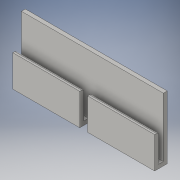
# Autodesk Inventor part: Handles
Saved by Autodesk Inventor 2016 (Build 200138000, 138)
## iProperties
Created: 2017-03-11
Part Number: Handles
Material: Generic
Document SubType Name: Modeling
Designer: RoboticsUser
Density: 1 g/cm^3
Appearance: Default
Author: RoboticsUser
Autodesk Inventor part; units mm, degrees
ref_plane "YZ Plane" through (0, 0, 0) normal (1, 0, 0) x (0, 1, 0)
ref_plane "XZ Plane" through (0, 0, 0) normal (0, 1, 0) x (-1, 0, 0)
ref_plane "XY Plane" through (0, 0, 0) normal (0, 0, 1) x (1, 0, 0)
sketch "Sketch5" plane through (0, 0, 0) normal (1, 0, 0) x (0, 1, 0)
  line L0 (0, 0) -> (101.6, 0)
  line L1 (101.6, 0) -> (101.6, -20.32)
  line L2 (101.6, -20.32) -> (0, -20.32)
  line L3 (0, -20.32) -> (0, 0)
  line L4 (101.6, -6.35) -> (6.35, -6.35)
  line L5 (6.35, -6.35) -> (6.35, -13.97)
  line L6 (6.35, -13.97) -> (101.6, -13.97)
  line L7 (101.6, -13.97) -> (101.6, -6.35)
  line L8 (101.6, 0) -> (50.8, 0)
  line L9 (50.8, -6.35) -> (101.6, -6.35)
  line L10 (101.6, -6.35) -> (101.6, 0)
  dimension "d26" = 101.6
  dimension "d27" = 20.32
  dimension "d28" = 95.25
  dimension "d29" = 7.62
  dimension "d30" = 6.35
  dimension "d31" = 50.8
  constraints: 22 end point, 5 parallel, 3 horizontal, 2 perpendicular, 2 point on line
  measures "d26" distance of L1.end L2.end
  measures "d27" distance of L0.end L1.end
  measures "d28" distance of L6.end L5.end
  measures "d29" distance of L4.end L5.end
  measures "d30" distance between parallel lines of L0 L4
  measures "d31" distance of L9.end L9.start
extrude "Extrusion4" add sketch "Sketch5" against normal blind 228.6
sketch "Sketch6" plane through (0, 0, 0) normal (1, 0, 0) x (0, 0, -1)
  line L0 (0, 101.6) -> (0, 0) projected
  line L1 (20.32, 0) -> (20.32, 101.6) projected
  line L2 (20.32, 101.6) -> (0, 101.6) projected
  line L3 (0, 0) -> (20.32, 0) projected
  line L4 (0, 101.6) -> (20.32, 101.6) projected
  line L5 (13.97, 101.6) -> (6.35, 101.6)
  line L6 (6.35, 101.6) -> (6.35, 6.35)
  line L7 (6.35, 6.35) -> (13.97, 6.35)
  line L8 (13.97, 6.35) -> (13.97, 101.6)
  line L9 (0, 0) -> (0, 101.6) projected
  line L10 (0, 101.6) -> (6.35, 101.6)
  line L11 (6.35, 101.6) -> (6.35, 50.8)
  line L12 (6.35, 50.8) -> (0, 50.8)
  line L13 (0, 50.8) -> (0, 101.6)
  dimension "d34" = 7.62
  dimension "d35" = 95.25
  dimension "d36" = 6.35
  dimension "d37" = 50.8
  constraints: 16 end point, 4 parallel, 2 horizontal, 2 perpendicular, 2 point on line
  measures "d34" distance of L7.end L6.end
  measures "d35" distance of L6.end L5.end
  measures "d36" distance between parallel lines of L0 L6
  measures "d37" distance between parallel lines of L3 L12
extrude "Extrusion5" cut sketch "Sketch6" against normal blind 228.6 contours L2 L8 L7 L6
sketch "Sketch7" plane through (0, 0, 0) normal (1, 0, 0) x (0, 0, -1)
  line L0 (6.35, 6.35) -> (6.35, 101.6) projected
  line L1 (6.35, 101.6) -> (0, 101.6) projected
  line L2 (0, 101.6) -> (0, 0) projected
  line L3 (0, 0) -> (20.32, 0) projected
  line L4 (20.32, 0) -> (20.32, 101.6) projected
  line L5 (20.32, 101.6) -> (13.97, 101.6) projected
  line L6 (13.97, 101.6) -> (13.97, 6.35) projected
  line L7 (13.97, 6.35) -> (6.35, 6.35) projected
  line L8 (0, 101.6) -> (0, 0) projected
  line L9 (6.35, 6.35) -> (6.35, 101.6) projected
  line L10 (0, 101.6) -> (3.175, 101.6)
  line L11 (6.35, 98.425) -> (6.35, 50.8)
  line L12 (6.35, 50.8) -> (0, 50.8)
  line L13 (0, 50.8) -> (0, 101.6)
  arc A0 (6.35, 98.425) -> (3.175, 101.6) centre (3.175, 98.425) ccw
  line L14 (0, 0) -> (20.32, 0) projected
  line L15 (0, 50.8) -> (3.175, 50.8)
  line L16 (6.35, 47.625) -> (6.35, 0)
  line L17 (6.35, 0) -> (0, 0)
  line L18 (0, 0) -> (0, 50.8)
  arc A1 (6.35, 47.625) -> (3.175, 50.8) centre (3.175, 47.625) ccw
  line L19 (6.35, 50.8) -> (6.35, 41.6275)
  dimension "d40" = 50.8
  dimension "d47" = 3.175
  dimension "d48" = 3.175
  constraints: 18 end point, 5 point on line, 4 parallel, 4 point on circle, 4 tangent, 2 centre point, 2 horizontal, 2 perpendicular
  measures "d40" distance between parallel lines of L3 L12
  measures "d47" radius of A0
  measures "d48" radius of A1
extrude "Extrusion6" cut sketch "Sketch7" against normal blind 228.6 contours A1 L12 L0 | L12 L2 L1 A0 L0 | A0 L1 L0
sketch "Sketch8" plane through (0, 50.8, 0) normal (0, 1, 0) x (1, 0, 0)
  line L0 (0, 13.97) -> (0, 6.35) projected
  line L1 (0, 13.97) -> (-228.6, 13.97) projected
  line L2 (-228.6, 6.35) -> (-228.6, 13.97) projected
  line L3 (0, 6.35) -> (-228.6, 6.35) projected
  line L4 (0, 3.175) -> (0, 0) projected
  line L5 (-228.6, 0) -> (-228.6, 3.175) projected
  line L6 (0, 0) -> (-228.6, 0) projected
  line L7 (-228.6, 13.97) -> (0, 13.97) projected
  line L8 (0, 20.32) -> (0, 13.97) projected
  line L9 (0, 20.32) -> (-228.6, 20.32) projected
  line L10 (-228.6, 13.97) -> (-228.6, 20.32) projected
  line L11 (-228.6, 13.97) -> (0, 13.97) projected
  line L12 (0, 0) -> (-228.6, 0) projected
  line L13 (0, 13.97) -> (-228.6, 13.97) projected
  line L14 (-107.95, 0) -> (-120.65, 0)
  line L15 (-120.65, 0) -> (-120.65, 13.97)
  line L16 (-120.65, 13.97) -> (-107.95, 13.97)
  line L17 (-107.95, 13.97) -> (-107.95, 0)
  line L18 (0, 3.175) -> (-228.6, 3.175) projected
  dimension "d43" = 12.7
  dimension "d44" = 107.95
  constraints: 8 end point, 2 parallel, 2 point on line, 1 horizontal, 1 perpendicular
  measures "d43" distance of L15.end L16.end
  measures "d44" distance between parallel lines of L4 L17
extrude "Extrusion7" cut sketch "Sketch8" against normal blind 228.6 contours L17 L3 L15 L1 | L17 L18 L15 L3 | L17 L6 L15 L18
body "Solid2"
